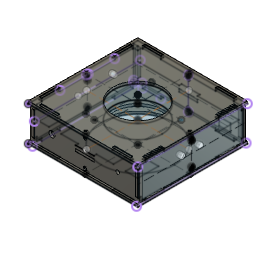
Magnetic-Stirrer (Autodesk Fusion 360 design; units mm, degrees)
Autodesk Fusion 360 part; units mm, degrees
(part 1 of 2)
sketch "Sketch1" plane through (0, 0, 0) normal (0, 1, 0) x (1, 0, 0) in component "floor"
  line L0 (0, 0) -> (180, 0)
  line L1 (180, 0) -> (180, 180)
  line L2 (180, 180) -> (0, 180)
  line L3 (0, 180) -> (0, 0)
  circle A0 centre (90, 90) radius 60
  line L4 (15, 177) -> (45, 177)
  line L5 (45, 177) -> (45, 173)
  line L6 (45, 173) -> (15, 173)
  line L7 (15, 173) -> (15, 177)
  line L8 (90, 180) -> (90, 0) construction
  line L9 (0, 90) -> (180, 90) construction
  line L10 (165, 173) -> (165, 177)
  line L11 (165, 177) -> (135, 177)
  line L12 (135, 173) -> (165, 173)
  line L13 (135, 177) -> (135, 173)
  line L14 (3, 165) -> (7, 165)
  line L15 (7, 165) -> (7, 135)
  line L16 (7, 135) -> (3, 135)
  line L17 (3, 135) -> (3, 165)
  line L18 (45, 7) -> (15, 7)
  line L19 (45, 3) -> (45, 7)
  line L20 (15, 7) -> (15, 3)
  line L21 (165, 7) -> (165, 3)
  line L22 (165, 3) -> (135, 3)
  line L23 (15, 3) -> (45, 3)
  line L24 (135, 7) -> (165, 7)
  line L25 (135, 3) -> (135, 7)
  line L26 (7, 15) -> (7, 45)
  line L27 (7, 45) -> (3, 45)
  line L28 (3, 45) -> (3, 15)
  line L29 (3, 15) -> (7, 15)
  line L30 (173, 135) -> (177, 135)
  line L31 (173, 45) -> (177, 45)
  line L32 (177, 15) -> (173, 15)
  line L33 (177, 135) -> (177, 165)
  line L34 (173, 165) -> (173, 135)
  line L35 (177, 165) -> (173, 165)
  line L36 (177, 45) -> (177, 15)
  line L37 (173, 15) -> (173, 45)
  circle A1 centre (90, 4.5) radius 1.5
  circle A2 centre (90, 175.5) radius 1.5
  circle A3 centre (175.5, 90) radius 1.5
  circle A4 centre (4.5, 90) radius 1.5
  dimension "d8" = 180
  dimension "d9" = 180
  dimension "d10" = 120
  dimension "d11" = 90
  dimension "d12" = 90
  dimension "d13" = 30
  dimension "d14" = 4
  dimension "d15" = 3
  dimension "d16" = 15
  dimension "d17" = 4
  dimension "d18" = 30
  dimension "d19" = 3
  dimension "d20" = 15
  dimension "d21" = 3
  dimension "d22" = 4.5
  dimension "d150" = 3
  dimension "d151" = 4.5
  dimension "d152" = 3
  dimension "d153" = 4.5
  constraint horizontal L0
  constraint vertical L1
  constraint horizontal L2
  constraint vertical L3
  constraint coincident L0.start L3.end
  constraint horizontal L4
  constraint vertical L5
  constraint horizontal L6
  constraint vertical L7
  constraint midpoint L2 L8.start
  constraint midpoint L0 L8.end
  constraint midpoint L3 L9.start
  constraint midpoint L1 L9.end
  constraint symmetric L4.start L8 L10.end
  constraint symmetric L4.end L8 L11.end
  constraint symmetric L5.end L8 L12.start
  constraint symmetric L6.end L8 L10.start
  constraint horizontal L14
  constraint vertical L15
  constraint horizontal L16
  constraint vertical L17
  constraint symmetric L4.start L9 L20.end
  constraint symmetric L4.end L9 L19.start
  constraint symmetric L5.end L9 L18.start
  constraint symmetric L6.end L9 L18.end
  constraint symmetric L9 L11.end L22.end
  constraint symmetric L9 L10.start L21.start
  constraint symmetric L9 L12.start L24.start
  constraint symmetric L9 L10.end L21.end
  constraint symmetric L9 L14.start L28.end
  constraint symmetric L9 L14.end L26.start
  constraint symmetric L9 L15.end L26.end
  constraint symmetric L9 L16.end L27.end
  constraint symmetric L8 L14.start L33.end
  constraint symmetric L8 L14.end L34.start
  constraint symmetric L8 L15.end L30.start
  constraint symmetric L8 L16.end L30.end
  constraint symmetric L8 L27.end L31.end
  constraint symmetric L8 L28.end L32.start
  constraint symmetric L8 L26.start L32.end
  constraint symmetric L8 L26.end L31.start
  constraint coincident L8 A1.centre
  constraint symmetric L9 A1 A2
  constraint coincident L9 A3.centre
  constraint coincident L9 A4.centre
  measures "d8" distance of L0.start L0.end
  measures "d9" distance of L0.start L2.end
  measures "d10" diameter of A0
  measures "d11" distance of L0 A0.centre
  measures "d12" distance of L1 A0.centre
  measures "d13" distance of L4.start L4.end
  measures "d14" distance of L4.start L6.end
  measures "d15" distance of L2 L4
  measures "d16" distance of L3 L7
  measures "d17" distance of L14.start L14.end
  measures "d18" distance of L14.start L16.end
  measures "d19" distance of L3 L17
  measures "d20" distance of L2 L14
  measures "d21" diameter of A1
  measures "d22" distance of L0 A1.centre
  measures "d150" diameter of A3
  measures "d151" distance of L1 A3.centre
  measures "d152" diameter of A4
  measures "d153" distance of L3 A4.centre
extrude "Extrude1" add sketch "Sketch1" along normal blind 4 contours L0 L1 L2 L3 | A3 | A4 makes body 1 in component "floor"
sketch "Sketch2" plane through (0, 0, 0) normal (0, 0, 1) x (1, 0, 0) in component "floor"
ref_plane "WorkPlane1" through (0, 0, -3) normal (0, 0, 1) x (1, 0, 0) in component "front"
sketch "Sketch1 (2)" plane through (0, 0, -3) normal (0, 0, 1) x (1, 0, 0) in component "front"
  line L0 (180, 56) -> (180, 4)
  line L1 (0, 4) -> (0, 56)
  line L2 (45, 4) -> (45, 0)
  line L3 (45, 0) -> (15, 0)
  line L4 (15, 0) -> (15, 4)
  line L5 (0, 0) -> (0, 4)
  line L6 (15, 4) -> (0, 4)
  line L7 (90, 56) -> (90, 4) construction
  line L8 (135, 4) -> (135, 0)
  line L9 (165, 0) -> (165, 4)
  line L10 (135, 0) -> (165, 0)
  line L11 (180, 4) -> (165, 4)
  line L12 (0, 30) -> (180, 30) construction
  line L13 (15, 60) -> (15, 56)
  line L14 (45, 56) -> (45, 60)
  line L15 (45, 60) -> (15, 60)
  line L16 (165, 60) -> (165, 56)
  line L17 (135, 56) -> (135, 60)
  line L18 (135, 60) -> (165, 60)
  line L19 (0, 56) -> (15, 56)
  line L20 (165, 56) -> (180, 56)
  circle A0 centre (36, 30) radius 5
  line L21 (75, 29) -> (105, 29)
  line L22 (105, 29) -> (105, 25)
  line L23 (105, 25) -> (75, 25)
  line L24 (75, 25) -> (75, 29)
  line L25 (3, 50) -> (7, 50)
  line L26 (7, 50) -> (7, 10)
  line L27 (7, 10) -> (3, 10)
  line L28 (3, 10) -> (3, 50)
  line L29 (173, 50) -> (173, 10)
  line L30 (177, 10) -> (177, 50)
  line L31 (173, 10) -> (177, 10)
  line L32 (177, 50) -> (173, 50)
  line L33 (91.5, 56) -> (91.5, 53)
  line L34 (91.5, 53) -> (92.75, 53)
  line L35 (92.75, 53) -> (92.75, 50.5)
  line L36 (92.75, 50.5) -> (91.5, 50.5)
  line L37 (91.5, 50.5) -> (91.5, 49)
  line L38 (91.5, 49) -> (88.5, 49)
  line L39 (88.5, 49) -> (88.5, 50.5)
  line L40 (88.5, 50.5) -> (87.25, 50.5)
  line L41 (87.25, 50.5) -> (87.25, 53)
  line L42 (87.25, 53) -> (88.5, 53)
  line L43 (88.5, 53) -> (88.5, 56)
  line L44 (91.5, 11) -> (88.5, 11)
  line L45 (91.5, 7) -> (92.75, 7)
  line L46 (87.25, 9.5) -> (87.25, 7)
  line L47 (92.75, 9.5) -> (91.5, 9.5)
  line L48 (91.5, 9.5) -> (91.5, 11)
  line L49 (88.5, 11) -> (88.5, 9.5)
  line L50 (92.75, 7) -> (92.75, 9.5)
  line L51 (88.5, 9.5) -> (87.25, 9.5)
  line L52 (87.25, 7) -> (88.5, 7)
  line L53 (91.5, 4) -> (91.5, 7)
  line L54 (88.5, 7) -> (88.5, 4)
  line L55 (45, 56) -> (88.5, 56)
  line L56 (91.5, 56) -> (135, 56)
  line L57 (135, 4) -> (91.5, 4)
  line L58 (88.5, 4) -> (45, 4)
  circle A1 centre (144, 30) radius 3
  dimension "d26" = 52
  dimension "d27" = 180
  dimension "d28" = 4
  dimension "d29" = 30
  dimension "d30" = 4
  dimension "d31" = 15
  dimension "d33" = 90
  dimension "d35" = 10
  dimension "d36" = 30
  dimension "d37" = 36
  dimension "d39" = 30
  dimension "d40" = 4
  dimension "d41" = 75
  dimension "d42" = 27
  dimension "d59" = 4
  dimension "d60" = 40
  dimension "d61" = 3
  dimension "d63" = 10
  dimension "d168" = 3
  dimension "d169" = 1.25
  dimension "d170" = 2.5
  dimension "d171" = 1.25
  dimension "d172" = 3
  dimension "d173" = 1.25
  dimension "d174" = 2.5
  dimension "d175" = 1.25
  dimension "d176" = 3
  dimension "d177" = 88.5
  dimension "d179" = 1.5
  dimension "d192" = 6
  dimension "d193" = 36
  constraint horizontal L19
  constraint vertical L0
  constraint horizontal L11
  constraint vertical L1
  constraint coincident L1 L5.start
  constraint vertical L2
  constraint horizontal L3
  constraint vertical L4
  constraint coincident L4.end L11
  constraint collinear L6 L11
  constraint coincident L7.end L11
  constraint perpendicular L7 L11
  constraint symmetric L4.end L7 L9.end
  constraint symmetric L2.start L7 L8.start
  constraint symmetric L2.end L7 L8.end
  constraint symmetric L3.end L7 L9.start
  constraint collinear L11 L57
  constraint midpoint L1 L12.start
  constraint midpoint L0 L12.end
  constraint symmetric L4.end L12 L13.end
  constraint symmetric L2.start L12 L14.start
  constraint symmetric L2.end L12 L14.end
  constraint symmetric L3.end L12 L13.start
  constraint symmetric L9.end L12 L16.end
  constraint symmetric L9.start L12 L16.start
  constraint symmetric L8.end L12 L17.end
  constraint symmetric L8.start L12 L17.start
  constraint collinear L19 L55
  constraint coincident L7.start L19
  constraint collinear L20 L55
  constraint horizontal L21
  constraint vertical L22
  constraint horizontal L23
  constraint vertical L24
  constraint horizontal L25
  constraint vertical L26
  constraint horizontal L27
  constraint vertical L28
  constraint symmetric L7 L25.start L30.end
  constraint symmetric L7 L25.end L29.start
  constraint symmetric L7 L26.end L29.end
  constraint symmetric L7 L27.end L30.start
  constraint coincident L33.start L55
  constraint perpendicular L33 L55
  constraint perpendicular L7 L34
  constraint perpendicular L34 L35
  constraint perpendicular L7 L36
  constraint perpendicular L36 L37
  constraint perpendicular L7 L38
  constraint perpendicular L36 L39
  constraint perpendicular L7 L40
  constraint perpendicular L40 L41
  constraint perpendicular L41 L42
  constraint perpendicular L43 L55
  constraint symmetric L12 L33.start L53.start
  constraint symmetric L12 L33.end L45.start
  constraint symmetric L12 L34.end L45.end
  constraint symmetric L12 L35.end L47.start
  constraint symmetric L12 L36.end L47.end
  constraint symmetric L12 L37.end L44.start
  constraint symmetric L12 L38.end L44.end
  constraint symmetric L12 L39.end L49.end
  constraint symmetric L12 L40.end L46.start
  constraint symmetric L12 L41.end L46.end
  constraint symmetric L12 L42.end L52.end
  constraint symmetric L12 L43.end L54.end
  constraint collinear L55 L56
  constraint collinear L57 L58
  constraint coincident L12 A1.centre
  measures "d26" distance of L1.end L1.start
  measures "d27" distance of L0 L1
  measures "d28" distance of L5.start L11
  measures "d29" distance of L4.end L2.start
  measures "d30" distance of L4.end L3.end
  measures "d31" distance of L4 L5
  measures "d33" distance of L1 L7
  measures "d35" diameter of A0
  measures "d36" distance of L3 A0.centre
  measures "d37" distance of L1 A0.centre
  measures "d39" distance of L21.start L21.end
  measures "d40" distance of L21.start L23.end
  measures "d41" distance of L1 L24
  measures "d42" distance of L21 L55
  measures "d59" distance of L25.start L25.end
  measures "d60" distance of L25.start L27.end
  measures "d61" distance of L1 L28
  measures "d63" distance of L3 L27
  measures "d168" distance of L33.start L33.end
  measures "d169" distance of L33.end L34.end
  measures "d170" distance of L34.end L35.end
  measures "d171" distance of L35.end L36.end
  measures "d172" distance of L37.end L38.end
  measures "d173" distance of L39.end L40.end
  measures "d174" distance of L40.end L41.end
  measures "d175" distance of L41.end L42.end
  measures "d176" distance of L42.end L43.end
  measures "d177" distance of L0 L33
  measures "d179" distance of L38 L40
  measures "d192" diameter of A1
  measures "d193" distance of L0 A1.centre
extrude "Extrude1'" add sketch "Sketch1 (2)" against normal blind 4 separate body contours L0 L1 L2 L3 L4 L6 L8 L9 L10 L11 L13 L14 L15 L16 L17 L18 L19 L20 L33 L34 L35 L36 L37 L38 L39 L40 L41 L42 L43 L44 L45 L46 L47 L48 L49 L50 L51 L52 L53 L54 L55 L56 L57 L58 | L25 L26 L27 L28 | L29 L30 L31 L32 | A1 makes body 2 in component "front"
ref_plane "WorkPlane1" through (0, 0, -173) normal (0, 0, 1) x (1, 0, 0) in component "back"
sketch "Sketch1 (3)" plane through (0, 0, -173) normal (0, 0, 1) x (1, 0, 0) in component "back"
  line L0 (180, 56) -> (180, 4)
  line L1 (0, 4) -> (0, 56)
  line L2 (45, 4) -> (45, 0)
  line L3 (45, 0) -> (15, 0)
  line L4 (15, 0) -> (15, 4)
  line L5 (0, 0) -> (0, 4)
  line L6 (15, 4) -> (0, 4)
  line L7 (90, 56) -> (90, 4) construction
  line L8 (135, 4) -> (135, 0)
  line L9 (165, 0) -> (165, 4)
  line L10 (135, 0) -> (165, 0)
  line L11 (180, 4) -> (165, 4)
  line L12 (0, 30) -> (180, 30) construction
  line L13 (15, 60) -> (15, 56)
  line L14 (45, 56) -> (45, 60)
  line L15 (45, 60) -> (15, 60)
  line L16 (165, 60) -> (165, 56)
  line L17 (135, 56) -> (135, 60)
  line L18 (135, 60) -> (165, 60)
  line L19 (0, 56) -> (15, 56)
  line L20 (165, 56) -> (180, 56)
  line L21 (75, 29) -> (105, 29)
  line L22 (105, 29) -> (105, 25)
  line L23 (105, 25) -> (75, 25)
  line L24 (75, 25) -> (75, 29)
  line L25 (140.6, 22.5) -> (159.4, 22.5)
  line L26 (159.4, 22.5) -> (159.4, 9.5)
  line L27 (159.4, 9.5) -> (140.6, 9.5)
  line L28 (140.6, 9.5) -> (140.6, 22.5)
  circle A0 centre (30, 16) radius 4
  line L29 (140.6, 16) -> (159.4, 16) construction
  line L30 (3, 50) -> (7, 50)
  line L31 (7, 50) -> (7, 10)
  line L32 (7, 10) -> (3, 10)
  line L33 (3, 10) -> (3, 50)
  line L34 (45, 0) -> (15, 0)
  line L35 (90, 56) -> (90, 4)
  line L36 (177, 10) -> (177, 50)
  line L37 (173, 50) -> (173, 10)
  line L38 (177, 50) -> (173, 50)
  line L39 (173, 10) -> (177, 10)
  line L40 (91.5, 56) -> (91.5, 53)
  line L41 (91.5, 53) -> (92.75, 53)
  line L42 (92.75, 53) -> (92.75, 50.5)
  line L43 (92.75, 50.5) -> (91.5, 50.5)
  line L44 (91.5, 50.5) -> (91.5, 49)
  line L45 (91.5, 49) -> (88.5, 49)
  line L46 (88.5, 49) -> (88.5, 50.5)
  line L47 (88.5, 50.5) -> (87.25, 50.5)
  line L48 (87.25, 50.5) -> (87.25, 53)
  line L49 (87.25, 53) -> (88.5, 53)
  line L50 (88.5, 53) -> (88.5, 56)
  line L51 (91.5, 7) -> (92.75, 7)
  line L52 (91.5, 9.5) -> (91.5, 11)
  line L53 (87.25, 7) -> (88.5, 7)
  line L54 (88.5, 11) -> (88.5, 9.5)
  line L55 (92.75, 7) -> (92.75, 9.5)
  line L56 (91.5, 11) -> (88.5, 11)
  line L57 (92.75, 9.5) -> (91.5, 9.5)
  line L58 (88.5, 7) -> (88.5, 4)
  line L59 (91.5, 4) -> (91.5, 7)
  line L60 (90, 4) -> (90, 56)
  line L61 (88.5, 9.5) -> (87.25, 9.5)
  line L62 (87.25, 9.5) -> (87.25, 7)
  line L63 (90, 4) -> (90, 56) construction
  line L64 (45, 56) -> (88.5, 56)
  line L65 (91.5, 56) -> (135, 56)
  line L66 (135, 4) -> (91.5, 4)
  line L67 (88.5, 4) -> (45, 4)
  dimension "d26_1" = 52
  dimension "d27_1" = 180
  dimension "d28_1" = 4
  dimension "d29_1" = 30
  dimension "d30_1" = 4
  dimension "d31_1" = 15
  dimension "d33_1" = 90
  dimension "d39_1" = 30
  dimension "d40_1" = 4
  dimension "d41_1" = 75
  dimension "d42_1" = 27
  dimension "d47" = 18.8
  dimension "d48" = 13
  dimension "d49" = 33.5
  dimension "d50" = 20.6
  dimension "d54" = 8
  dimension "d55" = 30
  dimension "d66" = 4
  dimension "d67" = 40
  dimension "d68" = 3
  dimension "d69" = 10
  dimension "d180" = 3
  dimension "d181" = 1.25
  dimension "d182" = 2.5
  dimension "d183" = 1.25
  dimension "d184" = 1.5
  dimension "d185" = 3
  dimension "d186" = 1.5
  dimension "d187" = 1.25
  dimension "d188" = 2.5
  dimension "d189" = 1.25
  dimension "d190" = 3
  dimension "d191" = 88.5
  constraint horizontal L19
  constraint vertical L0
  constraint horizontal L11
  constraint vertical L1
  constraint coincident L1 L5.start
  constraint vertical L2
  constraint horizontal L3
  constraint vertical L4
  constraint coincident L4.end L11
  constraint collinear L6 L11
  constraint coincident L7.end L11
  constraint perpendicular L7 L11
  constraint symmetric L4.end L7 L9.end
  constraint symmetric L2.start L7 L8.start
  constraint symmetric L2.end L7 L8.end
  constraint symmetric L3.end L7 L9.start
  constraint collinear L11 L66
  constraint midpoint L1 L12.start
  constraint midpoint L0 L12.end
  constraint symmetric L4.end L12 L13.end
  constraint symmetric L2.start L12 L14.start
  constraint symmetric L2.end L12 L14.end
  constraint symmetric L3.end L12 L13.start
  constraint symmetric L9.end L12 L16.end
  constraint symmetric L9.start L12 L16.start
  constraint symmetric L8.end L12 L17.end
  constraint symmetric L8.start L12 L17.start
  constraint collinear L19 L64
  constraint coincident L7.start L19
  constraint collinear L20 L64
  constraint horizontal L21
  constraint vertical L22
  constraint horizontal L23
  constraint vertical L24
  constraint horizontal L25
  constraint vertical L26
  constraint horizontal L27
  constraint vertical L28
  constraint midpoint L28 L29.start
  constraint midpoint L26 L29.end
  constraint coincident A0.centre L29
  constraint horizontal L30
  constraint vertical L31
  constraint horizontal L32
  constraint vertical L33
  constraint symmetric L30.start L35 L36.end
  constraint symmetric L30.end L35 L37.start
  constraint symmetric L31.end L35 L37.end
  constraint symmetric L32.end L35 L36.start
  constraint coincident L40.start L64
  constraint perpendicular L40 L64
  constraint perpendicular L7 L41
  constraint perpendicular L41 L42
  constraint perpendicular L35 L43
  constraint perpendicular L41 L44
  constraint perpendicular L7 L45
  constraint perpendicular L41 L46
  constraint perpendicular L7 L47
  constraint perpendicular L48 L64
  constraint perpendicular L7 L49
  constraint perpendicular L50 L64
  constraint symmetric L7.start L12 L7.end
  constraint symmetric L7.end L12 L7.start
  constraint symmetric L12 L7.start L7.end
  constraint symmetric L12 L7.end L7.start
  constraint symmetric L12 L40.start L59.start
  constraint symmetric L12 L40.end L51.start
  constraint symmetric L12 L41.end L51.end
  constraint symmetric L12 L42.end L55.end
  constraint symmetric L12 L43.end L52.start
  constraint symmetric L12 L44.end L52.end
  constraint symmetric L12 L45.end L54.start
  constraint symmetric L12 L46.end L54.end
  constraint symmetric L12 L47.end L61.end
  constraint symmetric L12 L48.end L53.start
  constraint symmetric L12 L49.end L53.end
  constraint symmetric L12 L50.end L58.end
  constraint collinear L64 L65
  constraint collinear L66 L67
  measures "d26_1" distance of L1.end L1.start
  measures "d27_1" distance of L0 L1
  measures "d28_1" distance of L5.start L11
  measures "d29_1" distance of L4.end L2.start
  measures "d30_1" distance of L4.end L3.end
  measures "d31_1" distance of L4 L5
  measures "d33_1" distance of L1 L7
  measures "d39_1" distance of L21.start L21.end
  measures "d40_1" distance of L21.start L23.end
  measures "d41_1" distance of L1 L24
  measures "d42_1" distance of L21 L64
  measures "d47" distance of L25.start L25.end
  measures "d48" distance of L25.start L27.end
  measures "d49" distance of L25 L64
  measures "d50" distance of L0 L26
  measures "d54" diameter of A0
  measures "d55" distance of L1 A0.centre
  measures "d66" distance of L30.start L30.end
  measures "d67" distance of L30.start L32.end
  measures "d68" distance of L1 L33
  measures "d69" distance of L32 L34
  measures "d180" distance of L40.start L40.end
  measures "d181" distance of L40.end L41.end
  measures "d182" distance of L41.end L42.end
  measures "d183" distance of L42.end L43.end
  measures "d184" distance of L43.end L44.end
  measures "d185" distance of L44.end L45.end
  measures "d186" distance of L45.end L46.end
  measures "d187" distance of L46.end L47.end
  measures "d188" distance of L47.end L48.end
  measures "d189" distance of L48.end L49.end
  measures "d190" distance of L49.end L50.end
  measures "d191" distance of L0 L40
extrude "Extrude1''" add sketch "Sketch1 (3)" against normal blind 4 separate body contours L0 L8 L9 L10 L11 L16 L17 L18 L20 L21 L22 L23 L35 L40 L41 L42 L43 L44 L45 L51 L52 L55 L56 L57 L59 L60 L65 L66 | L1 L2 L3 L4 L6 L13 L14 L15 L19 L21 L23 L24 L34 L35 L45 L46 L47 L48 L49 L50 L53 L54 L56 L58 L60 L61 L62 L64 L67 | L25 L26 L27 L28 | A0 | L30 L31 L32 L33 | L36 L37 L38 L39 makes body 3 in component "back"
extrude "Extrude2" cut sketch "Sketch1 (3)" against normal blind 10 contours L25 L26 L27 L28 bodies 3 in component "back"
extrude "Extrude3" cut sketch "Sketch1 (3)" against normal blind 15 contours L25 L26 L27 L28 | A0 bodies 3 in component "back"
extrude "Extrude2'" cut sketch "Sketch1 (2)" against normal blind 10 contours L25 L26 L27 L28 | L29 L30 L31 L32 bodies 2 in component "front"
ref_plane "WorkPlane1" through (7, 0, 0) normal (1, 0, 0) x (0, 1, 0) in component "left"
sketch "Sketch1 (4)" plane through (7, 0, 0) normal (1, 0, 0) x (0, 0, -1) in component "left"
  line L0 (173, 50) -> (177, 50)
  line L1 (177, 50) -> (177, 10)
  line L2 (177, 10) -> (173, 10)
  line L3 (180, 0) -> (0, 0)
  line L4 (173, 4) -> (173, 10)
  line L5 (173, 50) -> (173, 56)
  line L6 (90, 56) -> (90, 4) construction
  line L7 (3, 10) -> (7, 10)
  line L8 (7, 50) -> (3, 50)
  line L9 (3, 50) -> (3, 10)
  line L10 (7, 56) -> (7, 50)
  line L11 (7, 10) -> (7, 4)
  line L12 (135, 56) -> (135, 60)
  line L13 (135, 60) -> (165, 60)
  line L14 (165, 60) -> (165, 56)
  line L15 (173, 56) -> (165, 56)
  line L16 (45, 56) -> (45, 60)
  line L17 (15, 60) -> (15, 56)
  line L18 (45, 60) -> (15, 60)
  line L19 (15, 56) -> (7, 56)
  line L20 (177, 30) -> (3, 30) construction
  line L21 (135, 4) -> (135, 0)
  line L22 (135, 0) -> (165, 0)
  line L23 (165, 0) -> (165, 4)
  line L24 (45, 4) -> (45, 0)
  line L25 (15, 0) -> (15, 4)
  line L26 (45, 0) -> (15, 0)
  line L27 (165, 4) -> (173, 4)
  line L28 (7, 4) -> (15, 4)
  line L29 (91.5, 4) -> (91.5, 7)
  line L30 (91.5, 7) -> (92.75, 7)
  line L31 (92.75, 7) -> (92.75, 9.5)
  line L32 (92.75, 9.5) -> (91.5, 9.5)
  line L33 (91.5, 9.5) -> (91.5, 11)
  line L34 (91.5, 11) -> (90, 11)
  line L35 (87.25, 7) -> (87.25, 9.5)
  line L36 (88.5, 7) -> (87.25, 7)
  line L37 (87.25, 9.5) -> (88.5, 9.5)
  line L38 (88.5, 9.5) -> (88.5, 11)
  line L39 (88.5, 4) -> (88.5, 7)
  line L40 (88.5, 11) -> (90, 11)
  line L41 (92.75, 50.5) -> (91.5, 50.5)
  line L42 (88.5, 56) -> (88.5, 53)
  line L43 (91.5, 50.5) -> (91.5, 49)
  line L44 (88.5, 50.5) -> (88.5, 49)
  line L45 (88.5, 53) -> (87.25, 53)
  line L46 (92.75, 53) -> (92.75, 50.5)
  line L47 (87.25, 53) -> (87.25, 50.5)
  line L48 (91.5, 53) -> (92.75, 53)
  line L49 (87.25, 50.5) -> (88.5, 50.5)
  line L50 (91.5, 49) -> (90, 49)
  line L51 (88.5, 49) -> (90, 49)
  line L52 (91.5, 56) -> (91.5, 53)
  line L53 (135, 56) -> (91.5, 56)
  line L54 (88.5, 56) -> (45, 56)
  line L55 (45, 4) -> (88.5, 4)
  line L56 (91.5, 4) -> (135, 4)
  dimension "d80" = 166
  dimension "d81" = 52
  dimension "d82" = 7
  dimension "d83" = 4
  dimension "d84" = 4
  dimension "d85" = 40
  dimension "d86" = 10
  dimension "d87" = 30
  dimension "d88" = 4
  dimension "d89" = 12
  dimension "d92" = 3
  dimension "d93" = 1.25
  dimension "d95" = 2.5
  dimension "d96" = 1.25
  dimension "d97" = 1.5
  dimension "d99" = 1.5
  dimension "d100" = 1.5
  constraint horizontal L15
  constraint vertical L10
  constraint horizontal L28
  constraint vertical L4
  constraint horizontal L0
  constraint vertical L1
  constraint horizontal L2
  constraint coincident L0.start L4
  constraint collinear L4 L5
  constraint symmetric L0.start L6 L8.start
  constraint symmetric L0.end L6 L8.end
  constraint symmetric L1.end L6 L7.start
  constraint symmetric L2.end L6 L7.end
  constraint collinear L10 L11
  constraint vertical L12
  constraint horizontal L13
  constraint vertical L14
  constraint collinear L15 L53
  constraint coincident L6.start L15
  constraint symmetric L6 L14.end L17.end
  constraint symmetric L6 L12.start L16.start
  constraint symmetric L6 L12.end L16.end
  constraint symmetric L6 L13.end L17.start
  constraint collinear L19 L53
  constraint midpoint L1 L20.start
  constraint midpoint L9 L20.end
  constraint symmetric L14.end L20 L23.end
  constraint symmetric L12.start L20 L21.start
  constraint symmetric L12.end L20 L21.end
  constraint symmetric L13.end L20 L22.end
  constraint symmetric L16.start L20 L24.start
  constraint symmetric L17.start L20 L25.start
  constraint symmetric L17.end L20 L25.end
  constraint symmetric L16.end L20 L24.end
  constraint collinear L27 L28
  constraint coincident L6.end L28
  constraint collinear L28 L55
  constraint coincident L29.start L55
  constraint perpendicular L29 L55
  constraint perpendicular L6 L30
  constraint perpendicular L30 L31
  constraint perpendicular L6 L32
  constraint perpendicular L32 L33
  constraint perpendicular L6 L34
  constraint symmetric L6 L29.start L39.start
  constraint symmetric L6 L29.end L36.start
  constraint symmetric L6 L30.end L35.start
  constraint symmetric L6 L31.end L35.end
  constraint symmetric L6 L32.end L37.end
  constraint symmetric L6 L33.end L38.end
  constraint symmetric L6 L34.end L40.end
  constraint symmetric L20 L29.start L52.start
  constraint symmetric L20 L29.end L48.start
  constraint symmetric L20 L30.end L46.start
  constraint symmetric L20 L31.end L41.start
  constraint symmetric L20 L32.end L41.end
  constraint symmetric L20 L33.end L43.end
  constraint symmetric L20 L34.end L50.end
  constraint symmetric L20 L38.end L44.end
  constraint symmetric L20 L37.end L44.start
  constraint symmetric L20 L35.end L47.end
  constraint symmetric L20 L35.start L45.end
  constraint symmetric L20 L36.start L42.end
  constraint symmetric L20 L39.start L42.start
  constraint collinear L53 L54
  constraint collinear L55 L56
  measures "d80" distance of L5.end L10.start
  measures "d81" distance of L5.end L4.start
  measures "d82" distance of L3.end L10
  measures "d83" distance of L3.end L28
  measures "d84" distance of L0.start L0.end
  measures "d85" distance of L0.start L2.end
  measures "d86" distance of L2 L3
  measures "d87" distance of L14.end L12.start
  measures "d88" distance of L14.end L13.end
  measures "d89" distance of L1 L14
  measures "d92" distance of L29.start L29.end
  measures "d93" distance of L29.end L30.end
  measures "d95" distance of L30.end L31.end
  measures "d96" distance of L31.end L32.end
  measures "d97" distance of L32.end L33.end
  measures "d99" distance of L33.end L34.end
  measures "d100" distance of L6 L29
extrude "Extrude1'''" add sketch "Sketch1 (4)" against normal blind 4 separate body contours L0 L1 L2 L3 L4 L5 L7 L8 L9 L10 L11 L12 L13 L14 L15 L16 L17 L18 L19 L21 L22 L23 L24 L25 L26 L27 L28 L29 L30 L31 L32 L33 L34 L35 L36 L37 L38 L39 L40 L41 L42 L43 L44 L45 L46 L47 L48 L49 L50 L51 L52 L53 L54 L55 L56 makes body 4 in component "left"
move_body "Move1" bodies 3 to x (1, 0, 0) y (0, 1, 0) z (0, 0, 1) at (0, 0, -8) in component "back"
move_body "Move2" bodies 3 to x (1, 0, 0) y (0, 1, 0) z (0, 0, 1) at (0, 0, 8) in component "back"
ref_plane "WorkPlane1" through (7, 0, 0) normal (1, 0, 0) x (0, 1, 0) in component "right"
sketch "Sketch1 (5)" plane through (7, 0, 0) normal (1, 0, 0) x (0, 0, -1) in component "right"
  line L0 (173, 50) -> (177, 50)
  line L1 (177, 50) -> (177, 10)
  line L2 (177, 10) -> (173, 10)
  line L3 (180, 0) -> (0, 0)
  line L4 (173, 4) -> (173, 10)
  line L5 (173, 50) -> (173, 56)
  line L6 (90, 56) -> (90, 4) construction
  line L7 (3, 10) -> (7, 10)
  line L8 (7, 50) -> (3, 50)
  line L9 (3, 50) -> (3, 10)
  line L10 (7, 56) -> (7, 50)
  line L11 (7, 10) -> (7, 4)
  line L12 (135, 56) -> (135, 60)
  line L13 (135, 60) -> (165, 60)
  line L14 (165, 60) -> (165, 56)
  line L15 (173, 56) -> (165, 56)
  line L16 (45, 56) -> (45, 60)
  line L17 (15, 60) -> (15, 56)
  line L18 (45, 60) -> (15, 60)
  line L19 (15, 56) -> (7, 56)
  line L20 (177, 30) -> (3, 30) construction
  line L21 (135, 4) -> (135, 0)
  line L22 (135, 0) -> (165, 0)
  line L23 (165, 0) -> (165, 4)
  line L24 (45, 4) -> (45, 0)
  line L25 (15, 0) -> (15, 4)
  line L26 (45, 0) -> (15, 0)
  line L27 (165, 4) -> (173, 4)
  line L28 (7, 4) -> (15, 4)
  line L29 (91.5, 4) -> (91.5, 7)
  line L30 (91.5, 7) -> (92.75, 7)
  line L31 (92.75, 7) -> (92.75, 9.5)
  line L32 (92.75, 9.5) -> (91.5, 9.5)
  line L33 (91.5, 9.5) -> (91.5, 11)
  line L34 (91.5, 11) -> (90, 11)
  line L35 (87.25, 7) -> (87.25, 9.5)
  line L36 (88.5, 7) -> (87.25, 7)
  line L37 (87.25, 9.5) -> (88.5, 9.5)
  line L38 (88.5, 9.5) -> (88.5, 11)
  line L39 (88.5, 4) -> (88.5, 7)
  line L40 (88.5, 11) -> (90, 11)
  line L41 (92.75, 50.5) -> (91.5, 50.5)
  line L42 (88.5, 56) -> (88.5, 53)
  line L43 (91.5, 50.5) -> (91.5, 49)
  line L44 (88.5, 50.5) -> (88.5, 49)
  line L45 (88.5, 53) -> (87.25, 53)
  line L46 (92.75, 53) -> (92.75, 50.5)
  line L47 (87.25, 53) -> (87.25, 50.5)
  line L48 (91.5, 53) -> (92.75, 53)
  line L49 (87.25, 50.5) -> (88.5, 50.5)
  line L50 (91.5, 49) -> (90, 49)
  line L51 (88.5, 49) -> (90, 49)
  line L52 (91.5, 56) -> (91.5, 53)
  line L53 (135, 56) -> (91.5, 56)
  line L54 (88.5, 56) -> (45, 56)
  line L55 (45, 4) -> (88.5, 4)
  line L56 (91.5, 4) -> (135, 4)
  dimension "d80_1" = 166
  dimension "d81_1" = 52
  dimension "d82_1" = 7
  dimension "d83_1" = 4
  dimension "d84_1" = 4
  dimension "d85_1" = 40
  dimension "d86_1" = 10
  dimension "d87_1" = 30
  dimension "d88_1" = 4
  dimension "d89_1" = 12
  dimension "d92_1" = 3
  dimension "d93_1" = 1.25
  dimension "d95_1" = 2.5
  dimension "d96_1" = 1.25
  dimension "d97_1" = 1.5
  dimension "d99_1" = 1.5
  dimension "d100_1" = 1.5
  constraint horizontal L15
  constraint vertical L10
  constraint horizontal L28
  constraint vertical L4
  constraint horizontal L0
  constraint vertical L1
  constraint horizontal L2
  constraint coincident L0.start L4
  constraint collinear L4 L5
  constraint symmetric L0.start L6 L8.start
  constraint symmetric L0.end L6 L8.end
  constraint symmetric L1.end L6 L7.start
  constraint symmetric L2.end L6 L7.end
  constraint collinear L10 L11
  constraint vertical L12
  constraint horizontal L13
  constraint vertical L14
  constraint collinear L15 L53
  constraint coincident L6.start L15
  constraint symmetric L6 L14.end L17.end
  constraint symmetric L6 L12.start L16.start
  constraint symmetric L6 L12.end L16.end
  constraint symmetric L6 L13.end L17.start
  constraint collinear L19 L53
  constraint midpoint L1 L20.start
  constraint midpoint L9 L20.end
  constraint symmetric L14.end L20 L23.end
  constraint symmetric L12.start L20 L21.start
  constraint symmetric L12.end L20 L21.end
  constraint symmetric L13.end L20 L22.end
  constraint symmetric L16.start L20 L24.start
  constraint symmetric L17.start L20 L25.start
  constraint symmetric L17.end L20 L25.end
  constraint symmetric L16.end L20 L24.end
  constraint collinear L27 L28
  constraint coincident L6.end L28
  constraint collinear L28 L55
  constraint coincident L29.start L55
  constraint perpendicular L29 L55
  constraint perpendicular L6 L30
  constraint perpendicular L30 L31
  constraint perpendicular L6 L32
  constraint perpendicular L32 L33
  constraint perpendicular L6 L34
  constraint symmetric L6 L29.start L39.start
  constraint symmetric L6 L29.end L36.start
  constraint symmetric L6 L30.end L35.start
  constraint symmetric L6 L31.end L35.end
  constraint symmetric L6 L32.end L37.end
  constraint symmetric L6 L33.end L38.end
  constraint symmetric L6 L34.end L40.end
  constraint symmetric L20 L29.start L52.start
  constraint symmetric L20 L29.end L48.start
  constraint symmetric L20 L30.end L46.start
  constraint symmetric L20 L31.end L41.start
  constraint symmetric L20 L32.end L41.end
  constraint symmetric L20 L33.end L43.end
  constraint symmetric L20 L34.end L50.end
  constraint symmetric L20 L38.end L44.end
  constraint symmetric L20 L37.end L44.start
  constraint symmetric L20 L35.end L47.end
  constraint symmetric L20 L35.start L45.end
  constraint symmetric L20 L36.start L42.end
  constraint symmetric L20 L39.start L42.start
  constraint collinear L53 L54
  constraint collinear L55 L56
  measures "d80_1" distance of L5.end L10.start
  measures "d81_1" distance of L5.end L4.start
  measures "d82_1" distance of L3.end L10
  measures "d83_1" distance of L3.end L28
  measures "d84_1" distance of L0.start L0.end
  measures "d85_1" distance of L0.start L2.end
  measures "d86_1" distance of L2 L3
  measures "d87_1" distance of L14.end L12.start
  measures "d88_1" distance of L14.end L13.end
  measures "d89_1" distance of L1 L14
  measures "d92_1" distance of L29.start L29.end
  measures "d93_1" distance of L29.end L30.end
  measures "d95_1" distance of L30.end L31.end
  measures "d96_1" distance of L31.end L32.end
  measures "d97_1" distance of L32.end L33.end
  measures "d99_1" distance of L33.end L34.end
  measures "d100_1" distance of L6 L29
extrude "Extrude1''''" add sketch "Sketch1 (5)" against normal blind 4 separate body contours L0 L1 L2 L3 L4 L5 L7 L8 L9 L10 L11 L12 L13 L14 L15 L16 L17 L18 L19 L21 L22 L23 L24 L25 L26 L27 L28 L29 L30 L31 L32 L33 L34 L35 L36 L37 L38 L39 L40 L41 L42 L43 L44 L45 L46 L47 L48 L49 L50 L51 L52 L53 L54 L55 L56 makes body 5 in component "right"
sketch "Sketch1 (6)" plane through (0, 0, 0) normal (0, 1, 0) x (1, 0, 0) in component "top"
  line L0 (0, 0) -> (180, 0)
  line L1 (180, 0) -> (180, 180)
  line L2 (180, 180) -> (0, 180)
  line L3 (0, 180) -> (0, 0)
  circle A0 centre (90, 90) radius 40
  line L4 (15, 177) -> (45, 177)
  line L5 (45, 177) -> (45, 173)
  line L6 (45, 173) -> (15, 173)
  line L7 (15, 173) -> (15, 177)
  line L8 (90, 180) -> (90, 0) construction
  line L9 (0, 90) -> (180, 90) construction
  line L10 (165, 173) -> (165, 177)
  line L11 (165, 177) -> (135, 177)
  line L12 (135, 173) -> (165, 173)
  line L13 (135, 177) -> (135, 173)
  line L14 (3, 165) -> (7, 165)
  line L15 (7, 165) -> (7, 135)
  line L16 (7, 135) -> (3, 135)
  line L17 (3, 135) -> (3, 165)
  line L18 (45, 7) -> (15, 7)
  line L19 (45, 3) -> (45, 7)
  line L20 (15, 7) -> (15, 3)
  line L21 (165, 7) -> (165, 3)
  line L22 (165, 3) -> (135, 3)
  line L23 (15, 3) -> (45, 3)
  line L24 (135, 7) -> (165, 7)
  line L25 (135, 3) -> (135, 7)
  line L26 (7, 15) -> (7, 45)
  line L27 (7, 45) -> (3, 45)
  line L28 (3, 45) -> (3, 15)
  line L29 (3, 15) -> (7, 15)
  line L30 (173, 135) -> (177, 135)
  line L31 (173, 45) -> (177, 45)
  line L32 (177, 15) -> (173, 15)
  line L33 (177, 135) -> (177, 165)
  line L34 (173, 165) -> (173, 135)
  line L35 (177, 165) -> (173, 165)
  line L36 (177, 45) -> (177, 15)
  line L37 (173, 15) -> (173, 45)
  circle A1 centre (90, 4.5) radius 1.5
  circle A2 centre (90, 175.5) radius 1.5
  circle A3 centre (175.5, 90) radius 1.5
  line L38 (180, 0) -> (180, 180)
  line L39 (7, 88.5) -> (7, 45)
  circle A4 centre (5.5, 90) radius 1.5
  line L40 (7, 135) -> (7, 91.5)
  dimension "d8_1" = 180
  dimension "d9_1" = 180
  dimension "d10_1" = 80
  dimension "d11_1" = 90
  dimension "d12_1" = 90
  dimension "d13_1" = 30
  dimension "d14_1" = 4
  dimension "d15_1" = 3
  dimension "d16_1" = 15
  dimension "d17_1" = 4
  dimension "d18_1" = 30
  dimension "d19_1" = 3
  dimension "d20_1" = 15
  dimension "d21_1" = 3
  dimension "d22_1" = 4.5
  dimension "d158" = 3
  dimension "d159" = 4.5
  dimension "d162" = 3
  dimension "d163" = 1.5
  constraint horizontal L0
  constraint vertical L1
  constraint horizontal L2
  constraint vertical L3
  constraint coincident L0.start L3.end
  constraint horizontal L4
  constraint vertical L5
  constraint horizontal L6
  constraint vertical L7
  constraint midpoint L2 L8.start
  constraint midpoint L0 L8.end
  constraint midpoint L3 L9.start
  constraint midpoint L1 L9.end
  constraint symmetric L4.start L8 L10.end
  constraint symmetric L4.end L8 L11.end
  constraint symmetric L5.end L8 L12.start
  constraint symmetric L6.end L8 L10.start
  constraint horizontal L14
  constraint vertical L15
  constraint horizontal L16
  constraint vertical L17
  constraint symmetric L4.start L9 L20.end
  constraint symmetric L4.end L9 L19.start
  constraint symmetric L5.end L9 L18.start
  constraint symmetric L6.end L9 L18.end
  constraint symmetric L9 L11.end L22.end
  constraint symmetric L9 L10.start L21.start
  constraint symmetric L9 L12.start L24.start
  constraint symmetric L9 L10.end L21.end
  constraint symmetric L9 L14.start L28.end
  constraint symmetric L9 L14.end L26.start
  constraint symmetric L9 L15.end L26.end
  constraint symmetric L9 L16.end L27.end
  constraint symmetric L8 L14.start L33.end
  constraint symmetric L8 L14.end L34.start
  constraint symmetric L8 L15.end L30.start
  constraint symmetric L8 L16.end L30.end
  constraint symmetric L8 L27.end L31.end
  constraint symmetric L8 L28.end L32.start
  constraint symmetric L8 L26.start L32.end
  constraint symmetric L8 L26.end L31.start
  constraint coincident L8 A1.centre
  constraint symmetric L9 A1 A2
  constraint coincident L9 A3.centre
  constraint coincident L9 A4.centre
  measures "d8_1" distance of L0.start L0.end
  measures "d9_1" distance of L0.start L2.end
  measures "d10_1" diameter of A0
  measures "d11_1" distance of L0 A0.centre
  measures "d12_1" distance of L1 A0.centre
  measures "d13_1" distance of L4.start L4.end
  measures "d14_1" distance of L4.start L6.end
  measures "d15_1" distance of L2 L4
  measures "d16_1" distance of L3 L7
  measures "d17_1" distance of L14.start L14.end
  measures "d18_1" distance of L14.start L16.end
  measures "d19_1" distance of L3 L17
  measures "d20_1" distance of L2 L14
  measures "d21_1" diameter of A1
  measures "d22_1" distance of L0 A1.centre
  measures "d158" diameter of A3
  measures "d159" distance of A3.centre L38
  measures "d162" diameter of A4
  measures "d163" distance of A4.centre L40
extrude "Extrude1'''''" add sketch "Sketch1 (6)" along normal blind 4 separate body contours L0 L1 L2 L3 L38 | A3 | A4 makes body 6 in component "top"
sketch "Sketch2 (2)" plane through (0, 0, 0) normal (0, 0, 1) x (1, 0, 0) in component "top"
sketch "Sketch1 (7)" plane through (0, 0, 0) normal (0, 1, 0) x (1, 0, 0) in component "fan mount"
  line L0 (6, 135) -> (3, 135)
  line L1 (125.75, 54.25) -> (54.25, 54.25) construction
  line L2 (54.25, 54.25) -> (54.25, 125.75) construction
  line L3 (54.25, 125.75) -> (125.75, 125.75) construction
  line L4 (125.75, 125.75) -> (125.75, 54.25) construction
  circle A0 centre (54.25, 125.75) radius 1.5
  circle A1 centre (125.75, 125.75) radius 1.5
  circle A2 centre (125.75, 54.25) radius 1.5
  circle A3 centre (54.25, 54.25) radius 1.5
  circle A4 centre (90, 90) radius 40
  line L5 (174, 105) -> (177, 105)
  line L6 (177, 75) -> (174, 75)
  line L7 (105, 173) -> (105, 177)
  line L8 (105, 177) -> (75, 177)
  line L9 (75, 177) -> (75, 173)
  line L10 (90, 174) -> (90, 6) construction
  line L11 (6, 90) -> (174, 90) construction
  line L12 (105, 7) -> (105, 3)
  line L13 (105, 3) -> (75, 3)
  line L14 (75, 3) -> (75, 7)
  line L15 (7, 173) -> (75, 173)
  line L16 (105, 173) -> (173, 173)
  line L17 (7, 7) -> (7, 75)
  line L18 (7, 105) -> (7, 173)
  line L19 (173, 173) -> (173, 141)
  line L20 (173, 41) -> (173, 7)
  line L21 (173, 141) -> (153, 141)
  line L22 (153, 141) -> (153, 41)
  line L23 (153, 41) -> (173, 41)
  line L24 (47, 7) -> (47, 27)
  line L25 (47, 27) -> (27, 27)
  line L26 (27, 27) -> (27, 7)
  line L27 (7, 177) -> (7, 3)
  line L28 (153, 7) -> (153, 27)
  line L29 (153, 27) -> (133, 27)
  line L30 (133, 27) -> (133, 7)
  line L31 (173, 7) -> (153, 7)
  line L32 (133, 7) -> (105, 7)
  line L33 (75, 7) -> (47, 7)
  line L34 (27, 7) -> (7, 7)
  dimension "d104" = 71.5
  dimension "d105" = 71.5
  dimension "d108" = 3
  dimension "d110" = 3
  dimension "d111" = 3
  dimension "d114" = 166
  dimension "d115" = 166
  dimension "d116" = 7
  dimension "d117" = 7
  dimension "d118" = 47.25
  dimension "d119" = 47.25
  dimension "d120" = 80
  dimension "d121" = 90
  dimension "d122" = 90
  dimension "d123" = 30
  dimension "d125" = 68
  dimension "d126" = 30
  dimension "d127" = 4
  dimension "d128" = 68
  dimension "d130" = 30
  dimension "d132" = 30
  dimension "d133" = 4
  dimension "d134" = 68
  dimension "d136" = 20
  dimension "d137" = 100
  dimension "d138" = 34
  dimension "d139" = 20
  dimension "d140" = 20
  dimension "d141" = 20
  dimension "d142" = 20
  dimension "d143" = 20
  dimension "d144" = 20
  constraint horizontal L0
  constraint horizontal L1
  constraint vertical L2
  constraint horizontal L3
  constraint vertical L4
  constraint coincident L2.end L3.start
  constraint coincident L3.end L4.start
  constraint coincident L1.start L4.end
  constraint coincident L1.end L2.start
  constraint horizontal L15
  constraint vertical L19
  constraint horizontal L31
  constraint vertical L17
  constraint horizontal L5
  constraint horizontal L6
  constraint vertical L7
  constraint horizontal L8
  constraint vertical L9
  constraint coincident L18.start L17
  constraint vertical L12
  constraint horizontal L13
  constraint vertical L14
  constraint coincident L14.end L31
  constraint collinear L15 L16
  constraint collinear L17 L18
  constraint collinear L31 L33
  constraint collinear L19 L20
  constraint horizontal L21
  constraint vertical L22
  constraint horizontal L23
  constraint vertical L24
  constraint horizontal L25
  constraint vertical L26
  constraint coincident L26.end L33
  constraint vertical L28
  constraint horizontal L29
  constraint vertical L30
  constraint coincident L30.end L31
  constraint collinear L31 L32
  constraint collinear L33 L34
  measures "d104" distance of L1.start L1.end
  measures "d105" distance of L1.start L3.end
  measures "d108" diameter of A0
  measures "d110" diameter of A2
  measures "d111" diameter of A3
  measures "d114" distance of L15.start L17.start
  measures "d115" distance of L17 L19
  measures "d116" distance of origin L31
  measures "d117" distance of origin L17
  measures "d118" distance of L1 L31
  measures "d119" distance of L4 L19
  measures "d120" diameter of A4
  measures "d121" vertical distance of origin A4.centre
  measures "d122" horizontal distance of origin A4.centre
  measures "d123" distance of L5.start L6.end
  measures "d125" distance of L6 L31
  measures "d126" distance of L9.end L7.start
  measures "d127" distance of L9.end L8.end
  measures "d128" distance of L9 L17
  measures "d130" distance of L18.start L17.end
  measures "d132" distance of L14.end L12.start
  measures "d133" distance of L14.end L13.end
  measures "d134" distance of L14 L17
  measures "d136" distance of L19.end L21.end
  measures "d137" distance of L19.end L20.start
  measures "d138" distance of L23 L31
  measures "d139" distance of L26.end L24.start
  measures "d140" distance of L26.end L25.end
  measures "d141" distance of L26 L27
  measures "d142" distance of L30.end L28.start
  measures "d143" distance of L30.end L29.end
  measures "d144" distance of L20 L28
sketch "Sketch2 (3)" plane through (0, 0, 0) normal (0, 0, 1) x (1, 0, 0) in component "fan mount"
extrude "Extrude2''" add sketch "Sketch1 (7)" against normal blind 4 separate body makes body 7 in component "fan mount"
move_body "Move1'" bodies 7 to x (1, 0, 0) y (0, 1, 0) z (0, 0, 1) at (0, 5, 0) in component "fan mount"
move_body "Move2'" bodies 7 to x (1, 0, 0) y (0, 1, 0) z (0, 0, 1) at (0, -10, 0) in component "fan mount"
extrude "Extrude2'''" cut sketch "Sketch1" along normal blind 4 contours A4 bodies 1 in component "floor"
extrude "Extrude3'" cut sketch "Sketch1" along normal blind 4 contours A3 bodies 1 in component "floor"
extrude "Extrude2''''" cut sketch "Sketch1 (6)" along normal blind 4 contours A4 bodies 6 in component "top"
extrude "Extrude3''" cut sketch "Sketch1 (6)" along normal blind 4 contours A3 bodies 6 in component "top"
extrude "Extrude3'''" cut sketch "Sketch1 (2)" against normal blind 4 contours A1 bodies 2 in component "front"
component "floor" placed x (1, 0, 0) y (0, 1, 0) z (0, 0, 1) at (0, 0, 0)
component "front" placed x (1, 0, 0) y (0, 1, 0) z (0, 0, 1) at (0, 0, 0)
component "back" placed x (1, 0, 0) y (0, 1, 0) z (0, 0, 1) at (0, 0, 0)
component "left" placed x (1, 0, 0) y (0, 1, 0) z (0, 0, 1) at (171, 0, 0)
component "right" placed x (1, 0, 0) y (0, 1, 0) z (0, 0, 1) at (0, 0, 0)
component "top" placed x (1, 0, 0) y (0, 1, 0) z (0, 0, 1) at (0, 57, 0)
component "fan mount" placed x (1, 0, 0) y (0, 1, 0) z (0, 0, 1) at (0, 34, 0)
equation "total_width = 180 mm"
equation "total_length = 180 mm"
equation "total_height = 60 mm"
equation "material_thickness = 4 mm"
equation "bolt_size = 3 mm"
equation "wall_distance = 3 mm"
equation "fan_width = 80 mm"
equation "d8 = total_width"
equation "d9 = total_length"
equation "d10 = total_width / 1.5"
equation "d11 = total_length / 2"
equation "d12 = total_width / 2"
equation "d13 = total_width / 6"
equation "d14 = material_thickness"
equation "d15 = wall_distance"
equation "d16 = total_width / 12"
equation "d17 = material_thickness"
equation "d18 = total_length / 6"
equation "d19 = wall_distance"
equation "d20 = total_length / 12"
equation "d21 = bolt_size"
equation "d22 = wall_distance + ( bolt_size / 2 )"
equation "d23 = material_thickness"
equation "d25 = -wall_distance"
equation "d26 = total_height - ( material_thickness * 2 )"
equation "d27 = total_width"
equation "d28 = material_thickness"
equation "d29 = total_width / 6"
equation "d30 = material_thickness"
equation "d31 = total_width / 12"
equation "pot_holes = 6 mm"
equation "d36 = total_height / 2"
equation "d37 = total_width / 5"
equation "fan_height = 27 mm"
equation "d39 = total_width / 6"
equation "d40 = material_thickness"
equation "d41 = ( total_width / 2 ) - ( total_width / 12 )"
equation "d42 = fan_height"
equation "d43 = -material_thickness"
equation "d25_1 = -total_length + ( wall_distance + material_thickness )"
equation "d26_1 = total_height - ( material_thickness * 2 )"
equation "d27_1 = total_width"
equation "d28_1 = material_thickness"
equation "d29_1 = total_width / 6"
equation "d30_1 = material_thickness"
equation "d31_1 = total_width / 12"
equation "d39_1 = total_width / 6"
equation "d40_1 = material_thickness"
equation "d41_1 = ( total_width / 2 ) - ( total_width / 12 )"
equation "d42_1 = fan_height"
equation "d43_1 = -material_thickness"
equation "switch_width = 13 mm"
equation "switch_length = 18.8 mm"
equation "d47 = switch_length"
equation "d48 = switch_width"
equation "d49 = ( total_height * 2 / 3 ) - ( switch_width / 2 )"
equation "d50 = total_width / 6 - ( switch_length / 2 )"
equation "jack_diameter = 8 mm"
equation "d54 = jack_diameter"
equation "d55 = total_width / 6"
equation "d59 = material_thickness"
equation "d60 = total_height * ( 2 / 3 )"
equation "d61 = wall_distance"
equation "d63 = ( total_height - ( total_height * 2 / 3 ) ) / 2"
equation "d66 = material_thickness"
equation "d67 = total_height * 2 / 3"
equation "d68 = wall_distance"
equation "d69 = ( total_height - ( total_height * 2 / 3 ) ) / 2"
equation "d79 = wall_distance + material_thickness"
equation "d80 = total_length - ( material_thickness * 2 ) - ( wall_distance * 2 )"
equation "d81 = total_height - material_thickness * 2"
equation "d82 = wall_distance + material_thickness"
equation "d83 = material_thickness"
equation "d84 = material_thickness"
equation "d85 = total_height / 3 * 2"
equation "d86 = ( total_height - ( total_height * 2 / 3 ) ) / 2"
equation "d87 = total_length / 6"
equation "d88 = material_thickness"
equation "d89 = ( total_length / 12 ) - wall_distance"
equation "nut_width = 5.5 mm"
equation "bolt_depth = 3 mm"
equation "d92 = bolt_depth"
equation "d93 = ( nut_width - bolt_size ) / 2"
equation "nut_thickness = 2.5 mm"
equation "d95 = nut_thickness"
equation "d96 = ( nut_width - bolt_size ) / 2"
equation "d97 = bolt_depth / 2"
equation "d99 = bolt_size / 2"
equation "d100 = bolt_size / 2"
equation "d101 = -material_thickness"
equation "d79_1 = wall_distance + material_thickness"
equation "d80_1 = total_length - ( material_thickness * 2 ) - ( wall_distance * 2 )"
equation "d81_1 = total_height - material_thickness * 2"
equation "d82_1 = wall_distance + material_thickness"
equation "d83_1 = material_thickness"
equation "d84_1 = material_thickness"
equation "d85_1 = total_height / 3 * 2"
equation "d86_1 = ( total_height - ( total_height * 2 / 3 ) ) / 2"
equation "d87_1 = total_length / 6"
equation "d88_1 = material_thickness"
equation "d89_1 = total_length / 12 - wall_distance"
equation "d92_1 = bolt_depth"
equation "d93_1 = ( nut_width - bolt_size ) / 2"
equation "d95_1 = nut_thickness"
equation "d96_1 = ( nut_width - bolt_size ) / 2"
equation "d97_1 = bolt_depth / 2"
equation "d99_1 = bolt_size / 2"
equation "d100_1 = bolt_size / 2"
equation "d101_1 = -material_thickness"
equation "d8_1 = total_width"
equation "d9_1 = total_length"
equation "d11_1 = total_length / 2"
equation "d12_1 = total_width / 2"
equation "d13_1 = total_width / 6"
equation "d14_1 = material_thickness"
equation "d15_1 = wall_distance"
equation "d16_1 = total_width / 12"
equation "d17_1 = material_thickness"
equation "d18_1 = total_length / 6"
equation "d19_1 = wall_distance"
equation "d20_1 = total_length / 12"
equation "d21_1 = bolt_size"
equation "d22_1 = wall_distance + ( bolt_size / 2 )"
equation "d23_1 = material_thickness"
equation "fan_bolt_width = 71.5 mm"
equation "d104 = fan_bolt_width"
equation "d105 = fan_bolt_width"
equation "d108 = bolt_size"
equation "d110 = bolt_size"
equation "d111 = bolt_size"
equation "fan_hole_diameter = 80 mm"
equation "d114 = total_length - ( 2 * material_thickness ) - ( 2 * wall_distance )"
equation "d115 = total_width - ( 2 * wall_distance ) - ( 2 * material_thickness )"
equation "d116 = wall_distance + material_thickness"
equation "d117 = material_thickness + wall_distance"
equation "d118 = ( total_length - fan_bolt_width ) / 2 - material_thickness - wall_distance"
equation "d119 = ( total_width - fan_bolt_width ) / 2 - material_thickness - wall_distance"
equation "d120 = fan_hole_diameter"
equation "d121 = total_length / 2"
equation "d122 = total_width / 2"
equation "d123 = total_length / 6"